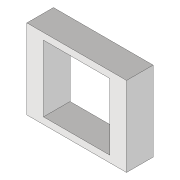
# Autodesk Inventor part: Grundkoerper
Saved by Autodesk Inventor 2020 (Build 240168000, 168)
## iProperties
Created: 2020-03-19
Part Number: Grundkoerper
Material: Generisch
Document SubType Name: Modeling
Designer: franz
Density: 1 g/cm^3
Appearance: Vorgabe
Author: franz
Autodesk Inventor part; units mm, degrees
ref_plane "YZ Plane" through (0, 0, 0) normal (1, 0, 0) x (0, 1, 0)
ref_plane "XZ Plane" through (0, 0, 0) normal (0, 1, 0) x (-1, 0, 0)
ref_plane "XY Plane" through (0, 0, 0) normal (0, 0, 1) x (1, 0, 0)
sketch "Skizze1" plane through (0, 0, 0) normal (0, 0, 1) x (1, 0, 0)
  line L0 (-50, -50) -> (50, -50)
  line L1 (50, -50) -> (50, 50)
  line L2 (50, 50) -> (-50, 50)
  line L3 (-50, 50) -> (-50, -50)
  line L4 (-50, -50) -> (50, 50) construction
  line L5 (50, -50) -> (-50, 50) construction
  line L6 (-75, -60) -> (75, -60)
  line L7 (75, -60) -> (75, 60)
  line L8 (75, 60) -> (-75, 60)
  line L9 (-75, 60) -> (-75, -60)
  line L10 (-75, -60) -> (75, 60) construction
  line L11 (75, -60) -> (-75, 60) construction
  point P0 (0, 0)
  dimension "d0" = 100
  dimension "d1" = 100
  dimension "d2" = 150
  dimension "d3" = 120
  constraints: 24 end point, 4 midpoint, 4 parallel, 2 horizontal, 2 perpendicular
  measures "d0" distance of L2.end L1.end
  measures "d1" distance of L1.end L0.end
  measures "d2" distance of L8.end L7.end
  measures "d3" distance of L7.end L6.end
extrude "Extrusion1" add sketch "Skizze1" along normal blind 40
sketch "Skizze2" plane through (-75, 60, 0) normal (0, 1, 0) x (1, 0, 0)
  circle A0 centre (140, -20) radius 5
  circle A1 centre (10, -20) radius 5
  line L0 (150, 0) -> (150, -40) projected
  line L1 (0, 0) -> (0, -40) projected
  line L2 (150, 0) -> (0, 0) projected
  line L3 (150, -40) -> (0, -40) projected
  point P0 (75, 0)
  dimension "d6" = 10
  dimension "d7" = 10
  dimension "d8" = 10
  dimension "d9" = 10
  dimension "d10" = 40
  dimension "d11" = 20
  dimension "d12" = 20
  constraints: 2 centre point
  measures "d6" diameter of A0
  measures "d7" diameter of A1
  measures "d8" distance from line of L0 A0.centre
  measures "d9" distance from line of L1 A1.centre
  measures "d10" distance between parallel lines of L2 L3
  measures "d11" distance from line of L2 A0.centre
  measures "d12" distance from line of L2 A1.centre
extrude "Extrusion2" cut sketch "Skizze2" against normal through all contours A0 | A1
equation "\"d7\" = d6"
equation "\"d9\" = d8"
equation "\"d11\" = 0.5 * d10"
equation "\"d12\" = d11"
